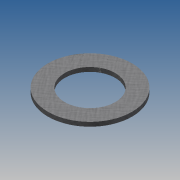
# Autodesk Inventor part: Distanzscheibe_6x10x0,5mm
Saved by Autodesk Inventor 2015 SP1 (Build 190203100, 203)
## iProperties
Created: 2015-02-20
Part Number: Distanzscheibe_6x10x0,5mm
Material: ABS-Kunststoff
Document SubType Name: Modeling
Designer: Marc
Mass: 0.0532814 g
Surface Area: 1.50796 cm^2
Volume: 0.0502655 cm^3
Density: 1.06 g/cm^3
Appearance: Gehont - dunkelgrau
Author: Marc
Autodesk Inventor part; units mm, degrees
ref_plane "YZ Plane" through (0, 0, 0) normal (1, 0, 0) x (0, 1, 0)
ref_plane "XZ Plane" through (0, 0, 0) normal (0, 1, 0) x (-1, 0, 0)
ref_plane "XY Plane" through (0, 0, 0) normal (0, 0, 1) x (1, 0, 0)
sketch "Skizze1" plane through (0, 0, 0) normal (0, 0, 1) x (1, 0, 0)
  line L0 (-7, 0) -> (7, 0) projected
  line L1 (0, -7) -> (0, 7) projected
  circle A0 centre (0, 0) radius 3
  circle A1 centre (0, 0) radius 5
  dimension "d0" = 6
  dimension "d1" = 10
  constraints: 2 centre point, 2 coincident
  measures "d0" diameter of A0
  measures "d1" diameter of A1
extrude "Extrusion1" add sketch "Skizze1" along normal blind 0.5 contours A0 L1 A1 L0 | L0 A1 L1 A0 | A0 L0 A1 L1 | L1 A1 L0 A0
